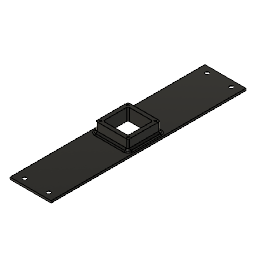
Overhead Stand Assembly (Autodesk Fusion 360 archive; units mm, degrees)
design "Camera Holder Middle"
Autodesk Fusion 360 part; units mm, degrees
sketch "Sketch1" plane through (0, 0, 0) normal (0, 0, 1) x (1, 0, 0)
  line L0 (-120.55, 25.4) -> (120.65, 25.4)
  line L1 (120.65, 25.4) -> (120.65, -25.4)
  line L2 (120.65, -25.4) -> (-120.55, -25.4)
  line L3 (-120.55, -25.4) -> (-120.55, 25.4)
  dimension "d3" = 241.2
  dimension "d4" = 50.8
  dimension "d5" = 25.4
  dimension "d6" = 120.65
  constraint horizontal L0
  constraint vertical L1
  constraint horizontal L2
  constraint vertical L3
  measures "d3" distance of L1 L3
  measures "d4" distance of L0 L2
  measures "d5" distance of origin L2
  measures "d6" distance of origin L1
extrude "Extrude1" add sketch "Sketch1" along normal blind 2.5
sketch "Sketch2" plane through (0, 0, 2.5) normal (0, 0, 1) x (-1, 0, 0)
  line L0 (120.55, 25.4) -> (-120.65, 25.4)
  line L1 (-120.65, 25.4) -> (-120.65, -25.4)
  line L2 (-120.65, -25.4) -> (120.55, -25.4)
  line L3 (120.55, -25.4) -> (120.55, 25.4)
  line L4 (13.4, -15.4) -> (-13.4, -15.4)
  line L5 (-15.4, -13.4) -> (-15.4, 13.4)
  line L6 (-13.4, 15.4) -> (13.4, 15.4)
  line L7 (15.4, 13.4) -> (15.4, -13.4)
  arc A0 (13.4, -15.4) -> (15.4, -13.4) centre (13.4, -13.4) ccw
  arc A1 (-15.4, -13.4) -> (-13.4, -15.4) centre (-13.4, -13.4) ccw
  arc A2 (-13.4, 15.4) -> (-15.4, 13.4) centre (-13.4, 13.4) ccw
  arc A3 (15.4, 13.4) -> (13.4, 15.4) centre (13.4, 13.4) ccw
  dimension "d7" = 30.8
  dimension "d8" = 30.8
  dimension "d9" = 15.4
  dimension "d10" = 15.4
  dimension "d11" = 2
  constraint horizontal L4
  constraint vertical L5
  constraint horizontal L6
  constraint vertical L7
  constraint tangent L4 A0
  constraint tangent L7 A0
  constraint tangent L4 A1
  constraint tangent L5 A1
  constraint equal A0 A1
  constraint tangent L5 A2
  constraint tangent L6 A2
  constraint equal A0 A2
  constraint tangent L6 A3
  constraint tangent L7 A3
  constraint equal A0 A3
  measures "d7" distance of L5 L7
  measures "d8" distance of L4 L6
  measures "d9" distance of origin L5
  measures "d10" distance of origin L4
  measures "d11" radius of A0
extrude "Extrude2" cut sketch "Sketch2" against normal blind 2.5 contours L4 L5 L6 L7 A0 A1 A2 A3
sketch "Sketch4" plane through (0, 0, 2.5) normal (0, 0, 1) x (-1, 0, 0)
  line L0 (15.4, 13.4) -> (15.4, -13.4)
  arc A0 (13.4, -15.4) -> (15.4, -13.4) centre (13.4, -13.4) ccw
  line L1 (13.4, -15.4) -> (-13.4, -15.4)
  arc A1 (-15.4, -13.4) -> (-13.4, -15.4) centre (-13.4, -13.4) ccw
  line L2 (-15.4, -13.4) -> (-15.4, 13.4)
  arc A2 (-13.4, 15.4) -> (-15.4, 13.4) centre (-13.4, 13.4) ccw
  line L3 (-13.4, 15.4) -> (13.4, 15.4)
  arc A3 (15.4, 13.4) -> (13.4, 15.4) centre (13.4, 13.4) ccw
  line L4 (120.55, 25.4) -> (-120.65, 25.4)
  line L5 (-120.65, 25.4) -> (-120.65, -25.4)
  line L6 (-120.65, -25.4) -> (120.55, -25.4)
  line L7 (120.55, -25.4) -> (120.55, 25.4)
  line L8 (18, -20) -> (-18, -20)
  line L9 (-20, -18) -> (-20, 18)
  line L10 (-18, 20) -> (18, 20)
  line L11 (20, 18) -> (20, -18)
  arc A4 (18, -20) -> (20, -18) centre (18, -18) ccw
  arc A5 (-20, -18) -> (-18, -20) centre (-18, -18) ccw
  arc A6 (-18, 20) -> (-20, 18) centre (-18, 18) ccw
  arc A7 (20, 18) -> (18, 20) centre (18, 18) ccw
  dimension "d18" = 40
  dimension "d19" = 40
  dimension "d20" = 20
  dimension "d21" = 20
  dimension "d22" = 2
  constraint horizontal L8
  constraint vertical L9
  constraint horizontal L10
  constraint vertical L11
  constraint tangent L8 A4
  constraint tangent L11 A4
  constraint tangent L8 A5
  constraint tangent L9 A5
  constraint equal A4 A5
  constraint tangent L9 A6
  constraint tangent L10 A6
  constraint equal A4 A6
  constraint tangent L10 A7
  constraint tangent L11 A7
  constraint equal A4 A7
  measures "d18" distance of L9 L11
  measures "d19" distance of L8 L10
  measures "d20" distance of origin L9
  measures "d21" distance of origin L8
  measures "d22" radius of A4
extrude "Extrude3" add sketch "Sketch4" along normal blind 2.5 contours L8 L9 L10 L11 A4 A5 A6 A7
sketch "Sketch6" plane through (0, 0, 5) normal (0, 0, 1) x (-1, 0, 0)
  arc A0 (13.4, -15.4) -> (15.4, -13.4) centre (13.4, -13.4) ccw
  line L0 (13.4, -15.4) -> (-13.4, -15.4)
  arc A1 (-15.4, -13.4) -> (-13.4, -15.4) centre (-13.4, -13.4) ccw
  line L1 (-15.4, -13.4) -> (-15.4, 13.4)
  arc A2 (-13.4, 15.4) -> (-15.4, 13.4) centre (-13.4, 13.4) ccw
  line L2 (-13.4, 15.4) -> (13.4, 15.4)
  arc A3 (15.4, 13.4) -> (13.4, 15.4) centre (13.4, 13.4) ccw
  line L3 (15.4, 13.4) -> (15.4, -13.4)
  arc A4 (18, -20) -> (20, -18) centre (18, -18) ccw
  line L4 (20, -18) -> (20, 18)
  arc A5 (20, 18) -> (18, 20) centre (18, 18) ccw
  line L5 (18, 20) -> (-18, 20)
  arc A6 (-18, 20) -> (-20, 18) centre (-18, 18) ccw
  line L6 (-20, 18) -> (-20, -18)
  arc A7 (-20, -18) -> (-18, -20) centre (-18, -18) ccw
  line L7 (-18, -20) -> (18, -20)
  point P0 (17, -17)
  point P1 (-17, -17)
  point P2 (-17, 17)
  point P3 (17, 17)
  dimension "d29" = 34
  dimension "d30" = 34
  dimension "d31" = 17
  dimension "d32" = 17
  constraint horizontal P0 P1
  constraint vertical P1 P2
  constraint horizontal P2 P3
  constraint vertical P0 P3
  measures "d29" horizontal distance of P0 P1
  measures "d30" vertical distance of P1 P2
  measures "d31" horizontal distance of origin P1
  measures "d32" vertical distance of origin P1
hole "Hole1" at (-17, 17, 5) at (17, 17, 5) at (17, -17, 5) at (-17, -17, 5) direction (0, 0, -1) diameter 2.54 depth 5 tip angle 118
chamfer "Chamfer1" distance 2.5 distance2 2.5 8 edges at (0, -20, 2.5) (-19.4142, -19.4142, 2.5) (-20, 0, 2.5) (-19.4142, 19.4142, 2.5) (0, 20, 2.5) (19.4142, 19.4142, 2.5) (20, 0, 2.5) (19.4142, -19.4142, 2.5) measured on face at (87.1, -6, 2.5) measured on face at (87.1, -6, 2.5) measured on face at (87.1, -6, 2.5) measured on face at (87.1, -6, 2.5) measured on face at (87.1, -6, 2.5) measured on face at (87.1, -6, 2.5) measured on face at (87.1, -6, 2.5) measured on face at (87.1, -6, 2.5)
fillet "Fillet1" radius 2.5 8 edges at (22.5, 0, 2.5) (21.182, 21.182, 2.5) (0, 22.5, 2.5) (-21.182, 21.182, 2.5) (-22.5, 0, 2.5) (-21.182, -21.182, 2.5) (0, -22.5, 2.5) (21.182, -21.182, 2.5)
sketch "Sketch7" plane through (0, 0, 0) normal (0, 0, -1) x (1, 0, 0)
  circle A0 centre (17, 17) radius 1.27
  circle A1 centre (-17, -17) radius 1.27
  circle A2 centre (17, -17) radius 1.27
  circle A3 centre (-17, 17) radius 1.27
  line L0 (-15.4, -13.4) -> (-15.4, 13.4)
  arc A4 (-13.4, 15.4) -> (-15.4, 13.4) centre (-13.4, 13.4) ccw
  line L1 (-13.4, 15.4) -> (13.4, 15.4)
  arc A5 (15.4, 13.4) -> (13.4, 15.4) centre (13.4, 13.4) ccw
  line L2 (15.4, 13.4) -> (15.4, -13.4)
  arc A6 (13.4, -15.4) -> (15.4, -13.4) centre (13.4, -13.4) ccw
  line L3 (13.4, -15.4) -> (-13.4, -15.4)
  arc A7 (-15.4, -13.4) -> (-13.4, -15.4) centre (-13.4, -13.4) ccw
  line L4 (120.65, 25.4) -> (-120.55, 25.4)
  line L5 (-120.55, 25.4) -> (-120.55, -25.4)
  line L6 (-120.55, -25.4) -> (120.65, -25.4)
  line L7 (120.65, -25.4) -> (120.65, 25.4)
  point P0 (-112.9, 15)
  point P1 (-112.9, -15)
  point P2 (113, 15)
  point P3 (113, -15)
  dimension "d40" = 30
  dimension "d41" = 7.65
  dimension "d42" = 7.65
  dimension "d48" = 10.4
  constraint horizontal P0 P2
  constraint vertical P2 P3
  constraint horizontal P1 P3
  constraint vertical P0 P1
  measures "d40" distance of P0 P1
  measures "d41" distance of L5 P0
  measures "d42" distance of L7 P2
  measures "d48" distance of L4 P0
hole "Hole2" at (-112.9, -15, 0) at (-112.9, 15, 0) at (113, -15, 0) at (113, 15, 0) direction (0, 0, 1) diameter 4.5 depth 5 tip angle 180 countersink diameter 9.4 countersink angle 90
extrude "Extrude5" add 9 faces at (6, 20, 4.9998) (-18.0952, 19.9977, 4.9997) (-17.0425, 4.4667, 5) (18.0952, 19.9977, 4.9998) (-20, -6, 4.9997) (20, 6, 4.9997) (-18.0952, -19.9977, 4.9998) (18.0952, -19.9977, 4.9997) (6, -20, 4.9997) along direction (0, 0, 1) blind 10
equation "d3 = 9.5 in - 0.1 mm"
equation "d6 = ( 9.5 / 2 ) * 1 in"
equation "d41 = ( ( 15.4 / 2 ) * 1 mm ) - 0.05 * 1 mm"
equation "d42 = ( ( 15.4 / 2 ) * 1 mm ) - 0.05 * 1 mm"
equation "d48 = ( 2 in - 30 mm ) / 2"

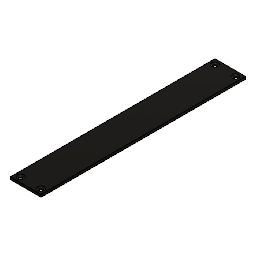
design "LED Light Holder Middle"
Autodesk Fusion 360 part; units mm, degrees
box "BoxPrimitive1" add length 200 width 30 height 5 placed x (0, 0, -1) y (-1, 0, 0) z (0, 1, 0) at (20, 0, 130) in component "Component"
sketch "Sketch2" plane through (0, 5, 0) normal (0, 1, 0) x (-1, 0, 0) in component "Component"
  line L0 (-20, -70) -> (10, -70)
  line L1 (10, -70) -> (10, 130)
  line L2 (10, 130) -> (-20, 130)
  line L3 (-20, 130) -> (-20, -70)
  point P0 (-15, -65)
  point P1 (5, -65)
  point P2 (-15, 125)
  point P3 (5, 125)
  dimension "d19" = 20
  dimension "d20" = 5
  dimension "d21" = 5
  dimension "d22" = 5
  constraint horizontal P2 P3
  constraint horizontal P0 P1
  constraint vertical P1 P3
  constraint vertical P0 P2
  measures "d19" distance of P2 P3
  measures "d20" distance of L3 P2
  measures "d21" distance of L2 P2
  measures "d22" distance of L0 P0
hole "Hole1" at (15, 5, -65) at (-5, 5, -65) at (-5, 5, 125) at (15, 5, 125) direction (0, -1, 0) diameter 3.4 depth 12 tip angle 118 countersink diameter 6.3 countersink angle 90 in component "Component"
extrude "Extrude1" cut 1 faces at (8.2675, 0, -1.0962) along direction (0, 1, 0) blind 2.5 in component "Component"
extrude "Extrude2" cut 1 faces at (8.2675, 2.5, -1.0962) along direction (0, 1, 0) blind 0.1 in component "Component"
component "Component" placed x (1, 0, 0) y (0, 1, 0) z (0, 0, 1) at (0, 0, 0)

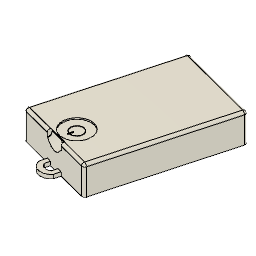
design "LED Light Battery Pack"
Autodesk Fusion 360 part; units mm, degrees
box "BoxPrimitive1" add length 103 width 64 height 22 placed x (0, 0, -1) y (-1, 0, 0) z (0, 1, 0) at (64, 0, 78) in component "Component"
sketch "Sketch2" plane through (0, 0, 0) normal (0, -1, 0) x (1, 0, 0) in component "Component"
  line L0 (0, -25) -> (64, -25)
  line L1 (64, -25) -> (64, 78)
  line L2 (64, 78) -> (0, 78)
  line L3 (0, 78) -> (0, -25)
  line L4 (39, -25) -> (24, -25)
  line L5 (24, -25) -> (24, -30)
  line L6 (24, -30) -> (39, -30)
  line L7 (39, -30) -> (39, -25)
  arc A0 (24, -30) -> (39, -30) centre (31.5, -26.9473) ccw
  constraint horizontal L4
  constraint vertical L5
  constraint horizontal L6
  constraint vertical L7
  constraint coincident L0 L4.start
extrude "Extrude1" add sketch "Sketch2" against normal blind 3 contours L0 L4 L5 L6 L7 | L6 A0 in component "Component"
sketch "Sketch3" plane through (0, 3, 0) normal (0, 1, 0) x (-1, 0, 0) in component "Component"
  arc A0 (-39, -30) -> (-24, -30) centre (-31.5, -26.9473) ccw
  line L0 (-24, -30) -> (-24, -25)
  line L1 (-24, -25) -> (-39, -25)
  line L2 (-39, -25) -> (-39, -30)
  line L3 (-27.5, -25) -> (-35.5, -25)
  line L4 (-35.5, -25) -> (-35.5, -29)
  line L5 (-35.5, -29) -> (-27.5, -29)
  line L6 (-27.5, -29) -> (-27.5, -25)
  arc A1 (-35.5, -29) -> (-27.5, -29) centre (-31.5, -26.0876) ccw
  constraint horizontal L3
  constraint vertical L4
  constraint horizontal L5
  constraint vertical L6
  constraint coincident L1 L3.start
extrude "Extrude2" cut sketch "Sketch3" against normal blind 5 contours L1 L3 L4 L5 L6 | L5 A1 in component "Component"
fillet "Fillet1" radius 2 1 edges at (0, 11, -25) in component "Component"
fillet "Fillet2" radius 2 1 edges at (0, 11, 78) in component "Component"
fillet "Fillet3" radius 2 1 edges at (64, 11, -25) in component "Component"
fillet "Fillet4" radius 2 1 edges at (64, 11, 78) in component "Component"
fillet "Fillet5" radius 2 8 edges at (0.5858, 22, 77.4142) (32, 22, 78) (63.4142, 22, 77.4142) (64, 22, 26.5) (63.4142, 22, -24.4142) (32, 22, -25) (0.5858, 22, -24.4142) (0, 22, 26.5) in component "Component"
sketch "Sketch1" plane through (0, 0, -25) normal (0, 0, -1) x (-1, 0, 0)
  line L0 (-2, 20) -> (-62, 20)
  line L1 (-62, 20) -> (-62, 0)
  line L2 (-62, 0) -> (-39, 0)
  line L3 (-39, 0) -> (-39, 3)
  line L4 (-39, 3) -> (-35.5, 3)
  line L5 (-35.5, 3) -> (-35.5, 0)
  line L6 (-35.5, 0) -> (-27.5, 0)
  line L7 (-27.5, 0) -> (-27.5, 3)
  line L8 (-27.5, 3) -> (-24, 3)
  line L9 (-24, 3) -> (-24, 0)
  line L10 (-24, 0) -> (-2, 0)
  line L11 (-2, 0) -> (-2, 20)
  circle A0 centre (-31.5187, 20) radius 7.4813
  constraint coincident L0 A0.centre
extrude "Extrude3" cut sketch "Sketch1" against normal blind 7 contours L0 A0 picked at (-33.0457, 17.6786) in component "Component"
pipe "Pipe1" cut diameter 6 along 1 edges at (31.5187, 20, -25) in component "Component"
sketch "Sketch2 (2)" plane through (0, 22, 0) normal (0, 1, 0) x (-1, 0, 0)
  line L0 (-2, 76) -> (-62, 76)
  line L1 (-62, 76) -> (-62, -23)
  line L2 (-24.0374, -23) -> (-2, -23)
  line L3 (-2, -23) -> (-2, 76)
  circle A0 centre (-31.0491, -11.1284) radius 11
  line L4 (-24.0374, -22.7639) -> (-24.0374, -23)
  line L5 (-62, -23) -> (-39, -23)
  line L6 (-39, -23) -> (-39, -22.7639)
  line L7 (-39, -22.7639) -> (-24.0374, -22.7639)
  dimension "d26" = 22
  measures "d26" diameter of A0
extrude "Extrude4" cut sketch "Sketch2 (2)" against normal blind 1 contours A0 in component "Component"
sketch "Sketch3 (2)" plane through (0, 21, 0) normal (0, 1, 0) x (-1, 0, 0)
  line L0 (-31.0491, -7.1059) -> (-31.0491, -15.1509) construction
  arc A0 (-30.1997, -15.9733) -> (-31.8985, -15.9733) centre (-31.0491, -11.1284) ccw
  arc A1 (-30.1997, -15.6907) -> (-31.8985, -15.6907) centre (-31.0491, -11.1284) ccw
  line L1 (-30.6514, -16.8752) -> (-30.6514, -13.4267)
  arc A2 (-30.6514, -13.4267) -> (-31.4468, -13.4267) centre (-31.0491, -13.4267) ccw
  line L2 (-31.4468, -13.4267) -> (-31.4468, -16.8752)
  arc A3 (-31.4468, -16.8752) -> (-30.6514, -16.8752) centre (-31.0491, -16.8752) ccw
  line L3 (-31.0491, -16.8752) -> (-31.0491, -13.4267) construction
  line L4 (-31.8985, -15.6907) -> (-31.8985, -15.9733)
  line L5 (-30.1997, -15.6907) -> (-30.1997, -15.9733)
  circle A4 centre (-31.0491, -11.1284) radius 11
  point P0 (-31.0491, -11.1284)
  point P1 (-31.0491, -15.1509)
  constraint concentric A0 A4
  constraint vertical L0
  constraint coincident P0 A0.centre
  constraint midpoint L0 P0
  constraint concentric A0 A1
  constraint tangent L1 A2
  constraint tangent A2 L2
  constraint parallel L1 L2
  constraint tangent L2 A3
  constraint tangent L1 A3
  constraint coincident L0 A2.centre
  constraint parallel L0 L3
  constraint coincident P1 L0.end
  constraint midpoint L3 P1
  constraint vertical L4
  constraint parallel L1 L5
extrude "Extrude5" cut sketch "Sketch3 (2)" against normal blind 0.5 contours A0 A1 L4 L5 | L1 A2 L2 A3 in component "Component"
component "Component" placed x (1, 0, 0) y (0, 1, 0) z (0, 0, 1) at (0, 0, 0)

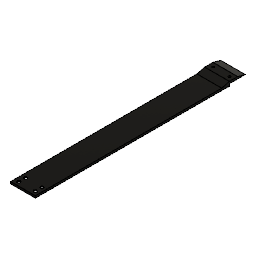
design "LED Light Holder Side"
Autodesk Fusion 360 part; units mm, degrees
form "Form1" [no effect] in component "Component"
box "BoxPrimitive1" add length 250 width 30 height -20 placed x (0, 0, -1) y (-1, 0, 0) z (0, 1, 0) at (30, 0, -100) in component "Component"
move_face "OffsetFaces1" offset -15 1 faces at (10, 0, -183.3333) in component "Component"
sketch "Sketch9" plane through (0, -20, 0) normal (0, -1, 0) x (1, 0, 0) in component "Component"
  line L0 (30, -100) -> (0, -100)
  line L1 (0, -100) -> (0, -350)
  line L2 (0, -350) -> (30, -350)
  line L3 (30, -350) -> (30, -100)
  point P0 (5, -120)
  point P1 (25, -120)
  point P2 (5, -128)
  point P3 (25, -128)
  dimension "d31" = 20
  dimension "d32" = 5
  dimension "d33" = 8
  dimension "d49" = 20
  constraint horizontal P0 P1
  constraint vertical P0 P2
  constraint horizontal P2 P3
  constraint vertical P1 P3
  measures "d31" distance of P0 P1
  measures "d32" distance of L1 P2
  measures "d33" distance of P0 P2
  measures "d49" distance of L0 P1
hole "Hole4" at (25, -20, -120) at (5, -20, -120) at (5, -20, -128) at (25, -20, -128) direction (0, 1, 0) diameter 3.797 depth 9 tip angle 180 countersink diameter 7.087 countersink angle 82 in component "Component"
extrude "Extrude4" cut 1 faces at (20, -18.3333, -350) along direction (0, 0, 1) blind 0.05 in component "Component"
extrude "Extrude5" cut 1 faces at (11.6667, -15, -276.5995) along direction (0, -1, 0) blind 2.5 in component "Component"
sketch "Sketch10" plane through (30, 0, 0) normal (1, 0, 0) x (0, 0, -1) in component "Component"
  line L0 (349.95, -17.5) -> (100, -17.5)
  line L1 (100, -17.5) -> (100, -20)
  line L2 (100, -20) -> (349.95, -20)
  line L3 (349.95, -20) -> (349.95, -17.5)
  line L4 (349.95, -17.5) -> (362.45, -17.5)
  line L5 (362.45, -17.5) -> (362.45, -15)
  line L6 (362.45, -15) -> (349.95, -15)
  line L7 (349.95, -15) -> (349.95, -17.5)
  line L8 (349.95, -15) -> (340.6199, -17.5)
  line L9 (362.45, -17.5) -> (372.45, -17.5)
  line L10 (359.95, -15) -> (369.2801, -17.5)
  dimension "d38" = 2.5
  dimension "d39" = 12.5
  dimension "d41" = 75
  dimension "d52" = 10
  dimension "d54" = 15
  dimension "d55" = 10
  constraint horizontal L4
  constraint vertical L5
  constraint horizontal L6
  constraint vertical L7
  constraint coincident L0 L3.end
  constraint vertical L2.end L6.end
  constraint coincident L0 L8.end
  constraint perpendicular L5 L9
  constraint coincident L6 L10.start
  constraint coincident L9 L10.end
  measures "d38" distance of L4 L6
  measures "d39" distance of L5 L7
  measures "d41" angle of L7 L8
  measures "d52" distance of L4.end L9.end
  measures "d54" angle of L6 L10
  measures "d55" distance of L6.end L10.start
extrude "Extrude6" add sketch "Sketch10" against normal blind 30 contours L4 L5 L6 L7 L10 | L0 L7 L8 | L5 L9 L10 in component "Component"
sketch "Sketch11" plane through (0, -15, 0) normal (0, 1, 0) x (-1, 0, 0) in component "Component"
  line L0 (-30, -349.95) -> (-30, -359.95)
  line L1 (0, -359.95) -> (0, -349.95)
  line L2 (0, -349.95) -> (-30, -349.95)
  line L3 (0, -349.95) -> (-30, -349.95)
  line L4 (-30, -359.95) -> (0, -359.95)
  point P0 (-5, -355)
  point P1 (-25, -355)
  dimension "d44" = 20
  dimension "d45" = 5
  dimension "d46" = 5.05
  constraint horizontal P0 P1
  measures "d44" distance of P0 P1
  measures "d45" distance of L0 P1
  measures "d46" distance of P1 L3
hole "Hole5" at (25, -15, -355) at (5, -15, -355) direction (0, -1, 0) diameter 2.85 end through all in component "Component"
extrude "Extrude7" cut 1 faces at (20, -19.1667, -100) along direction (0, 0, -1) blind 15 in component "Component"
component "Component" placed x (1, 0, 0) y (0, 1, 0) z (0, 0, 1) at (0, 0, 0)
